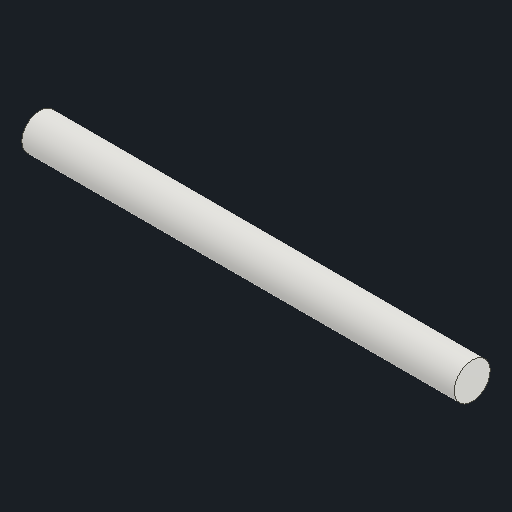
# Autodesk Inventor part: Shaft
Saved by Autodesk Inventor 2022 (Build 260153000, 153)
## iProperties
Created: 2021-12-02
Part Number: Shaft
Material: Steel
Document SubType Name: Modeling
Designer: izack
Density: 1 g/cm^3
Appearance: Steel
CustomPartVersion: 1
Author: izack
Length: 3.000 in
Autodesk Inventor part; units mm, degrees
ref_plane "Start Plane" through (0, 0, 0) normal (1, 0, 0) x (0, 1, 0)
ref_plane "XZ Plane" through (0, 0, 0) normal (0, 1, 0) x (-1, 0, 0)
ref_plane "XY Plane" through (0, 0, 0) normal (0, 0, 1) x (1, 0, 0)
sketch "Main Sketch" plane through (0, 0, 0) normal (0, 0, 1) x (1, 0, 0)
  line L0 (0, 0) -> (76.2, 0)
  line L1 (0, 0) -> (0, 3.175)
  line L2 (76.2, 3.175) -> (76.2, 0)
  line L3 (0, 3.175) -> (76.2, 3.175)
  constraints: 8 end point, 2 horizontal, 2 vertical
revolve "Revolution1" add sketch "Main Sketch" angle 360 about axis through (0, 0, 0) along (1, 0, 0)
equation "\"Length\" = 76.2"
body "Solid1"
